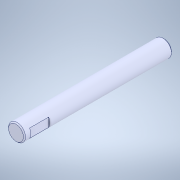
# Autodesk Inventor part: motor_antigravity_4004_custom_shaft
Saved by Autodesk Inventor 2022.2 (Build 262287030, 287C)
## iProperties
Created: 2016-08-15
Part Number: motor_antigravity_4004_custom_shaft
Material: SolidWorks DIN Materials|1.4000 (X6Cr13)
Document SubType Name: Modeling
Designer: Jochen
Density: 7.7 g/cm^3
Appearance: 202,209,238
Sending System: SolidWorks 2017
Last Author: Felix
Last Saved: 2019-07-15
Author: Jochen
Autodesk Inventor part; units mm, degrees
ref_plane "YZ Plane" through (0, 0, 0) normal (1, 0, 0) x (0, 1, 0)
ref_plane "XZ Plane" through (0, 0, 0) normal (0, 1, 0) x (-1, 0, 0)
ref_plane "XY Plane" through (0, 0, 0) normal (0, 0, 1) x (1, 0, 0)
sketch "Sketch1" plane through (0, 0, 0) normal (0, 0, 1) x (1, 0, 0)
  circle A0 centre (0, 0) radius 2
  dimension "d0" = 4
  constraints: 1 centre point, 1 coincident
  measures "d0" diameter of A0
extrude "Extrusion1" add sketch "Sketch1" along normal blind 34.9
chamfer "Chamfer1" distance 0.25 angle 45 2 edges at (-2, 0, 0) (-2, 0, 34.9)
sketch "Sketch3" plane through (0, 0, 0) normal (1, 0, 0) x (0, 1, 0)
  line L0 (2.5, 28.9) -> (-2.5, 28.9)
  line L1 (-2.5, 28.9) -> (-2.5, 33.4)
  line L2 (-2.5, 33.4) -> (2.5, 33.4)
  line L3 (2.5, 33.4) -> (2.5, 28.9)
  line L4 (-1.75, 34.9) -> (1.75, 34.9) projected
  line L5 (0, -6.9) -> (0, 41.4) construction
  point P0 (0, 0)
  dimension "d6" = 1.5
  dimension "d7" = 4.5
  dimension "d8" = 5
  constraints: 8 end point, 2 parallel, 1 horizontal, 1 perpendicular, 1 other
  measures "d6" distance between parallel lines of L4 L2
  measures "d7" distance of L0.end L1.end
  measures "d8" distance of L0.start L0.end
extrude "Extrusion2" add sketch "Sketch3" along normal mid plane 10 separate body
extrude "Extrusion3" cut sketch "Sketch3" along normal mid plane 3.4 bodies 2
combine bodies "Combine1" operation type subtract main body 1 bodies to subtract 2
body "Solid1"
body "Solid2"
